Autodesk Fusion 360 part; units mm, degrees
note: some values were not read from the file. Set by a fixed rule: which sketch regions a step uses.
(part 2 of 4)
  line L1067 (-99, -2.5) -> (-101, -2.5)
  line L1068 (-111, -5) -> (-109, -5)
  line L1069 (-109, -5) -> (-109, -2.5)
  line L1070 (-111, -2.5) -> (-111, -5)
  line L1071 (-109, -2.5) -> (-111, -2.5)
  line L1072 (-121, -5) -> (-119, -5)
  line L1073 (-119, -5) -> (-119, -2.5)
  line L1074 (-121, -2.5) -> (-121, -5)
  line L1075 (-119, -2.5) -> (-121, -2.5)
  line L1076 (-131, -5) -> (-129, -5)
  line L1077 (-129, -5) -> (-129, -2.5)
  line L1078 (-131, -2.5) -> (-131, -5)
  line L1079 (-129, -2.5) -> (-131, -2.5)
  line L1080 (-141, -5) -> (-139, -5)
  line L1081 (-139, -5) -> (-139, -2.5)
  line L1082 (-141, -2.5) -> (-141, -5)
  line L1083 (-139, -2.5) -> (-141, -2.5)
  line L1084 (-151, -5) -> (-149, -5)
  line L1085 (-149, -5) -> (-149, -2.5)
  line L1086 (-151, -2.5) -> (-151, -5)
  line L1087 (-149, -2.5) -> (-151, -2.5)
  line L1088 (-11, -15) -> (-9, -15)
  line L1089 (-9, -15) -> (-9, -12.5)
  line L1090 (-11, -12.5) -> (-11, -15)
  line L1091 (-9, -12.5) -> (-11, -12.5)
  line L1092 (-21, -15) -> (-19, -15)
  line L1093 (-19, -15) -> (-19, -12.5)
  line L1094 (-21, -12.5) -> (-21, -15)
  line L1095 (-19, -12.5) -> (-21, -12.5)
  line L1096 (-31, -15) -> (-29, -15)
  line L1097 (-29, -15) -> (-29, -12.5)
  line L1098 (-31, -12.5) -> (-31, -15)
  line L1099 (-29, -12.5) -> (-31, -12.5)
  line L1100 (-41, -15) -> (-39, -15)
  line L1101 (-39, -15) -> (-39, -12.5)
  line L1102 (-41, -12.5) -> (-41, -15)
  line L1103 (-39, -12.5) -> (-41, -12.5)
  line L1104 (-51, -15) -> (-49, -15)
  line L1105 (-49, -15) -> (-49, -12.5)
  line L1106 (-51, -12.5) -> (-51, -15)
  line L1107 (-49, -12.5) -> (-51, -12.5)
  line L1108 (-61, -15) -> (-59, -15)
  line L1109 (-59, -15) -> (-59, -12.5)
  line L1110 (-61, -12.5) -> (-61, -15)
  line L1111 (-59, -12.5) -> (-61, -12.5)
  line L1112 (-71, -15) -> (-69, -15)
  line L1113 (-69, -15) -> (-69, -12.5)
  line L1114 (-71, -12.5) -> (-71, -15)
  line L1115 (-69, -12.5) -> (-71, -12.5)
  line L1116 (-81, -15) -> (-79, -15)
  line L1117 (-79, -15) -> (-79, -12.5)
  line L1118 (-81, -12.5) -> (-81, -15)
  line L1119 (-79, -12.5) -> (-81, -12.5)
  line L1120 (-91, -15) -> (-89, -15)
  line L1121 (-89, -15) -> (-89, -12.5)
  line L1122 (-91, -12.5) -> (-91, -15)
  line L1123 (-89, -12.5) -> (-91, -12.5)
  line L1124 (-101, -15) -> (-99, -15)
  line L1125 (-99, -15) -> (-99, -12.5)
  line L1126 (-101, -12.5) -> (-101, -15)
  line L1127 (-99, -12.5) -> (-101, -12.5)
  line L1128 (-111, -15) -> (-109, -15)
  line L1129 (-109, -15) -> (-109, -12.5)
  line L1130 (-111, -12.5) -> (-111, -15)
  line L1131 (-109, -12.5) -> (-111, -12.5)
  line L1132 (-121, -15) -> (-119, -15)
  line L1133 (-119, -15) -> (-119, -12.5)
  line L1134 (-121, -12.5) -> (-121, -15)
  line L1135 (-119, -12.5) -> (-121, -12.5)
  line L1136 (-131, -15) -> (-129, -15)
  line L1137 (-129, -15) -> (-129, -12.5)
  line L1138 (-131, -12.5) -> (-131, -15)
  line L1139 (-129, -12.5) -> (-131, -12.5)
  line L1140 (-141, -15) -> (-139, -15)
  line L1141 (-139, -15) -> (-139, -12.5)
  line L1142 (-141, -12.5) -> (-141, -15)
  line L1143 (-139, -12.5) -> (-141, -12.5)
  line L1144 (-151, -15) -> (-149, -15)
  line L1145 (-149, -15) -> (-149, -12.5)
  line L1146 (-151, -12.5) -> (-151, -15)
  line L1147 (-149, -12.5) -> (-151, -12.5)
  line L1148 (-11, -25) -> (-9, -25)
  line L1149 (-9, -25) -> (-9, -22.5)
  line L1150 (-11, -22.5) -> (-11, -25)
  line L1151 (-9, -22.5) -> (-11, -22.5)
  line L1152 (-21, -25) -> (-19, -25)
  line L1153 (-19, -25) -> (-19, -22.5)
  line L1154 (-21, -22.5) -> (-21, -25)
  line L1155 (-19, -22.5) -> (-21, -22.5)
  line L1156 (-31, -25) -> (-29, -25)
  line L1157 (-29, -25) -> (-29, -22.5)
  line L1158 (-31, -22.5) -> (-31, -25)
  line L1159 (-29, -22.5) -> (-31, -22.5)
  line L1160 (-41, -25) -> (-39, -25)
  line L1161 (-39, -25) -> (-39, -22.5)
  line L1162 (-41, -22.5) -> (-41, -25)
  line L1163 (-39, -22.5) -> (-41, -22.5)
  line L1164 (-51, -25) -> (-49, -25)
  line L1165 (-49, -25) -> (-49, -22.5)
  line L1166 (-51, -22.5) -> (-51, -25)
  line L1167 (-49, -22.5) -> (-51, -22.5)
  line L1168 (-61, -25) -> (-59, -25)
  line L1169 (-59, -25) -> (-59, -22.5)
  line L1170 (-61, -22.5) -> (-61, -25)
  line L1171 (-59, -22.5) -> (-61, -22.5)
  line L1172 (-71, -25) -> (-69, -25)
  line L1173 (-69, -25) -> (-69, -22.5)
  line L1174 (-71, -22.5) -> (-71, -25)
  line L1175 (-69, -22.5) -> (-71, -22.5)
  line L1176 (-81, -25) -> (-79, -25)
  line L1177 (-79, -25) -> (-79, -22.5)
  line L1178 (-81, -22.5) -> (-81, -25)
  line L1179 (-79, -22.5) -> (-81, -22.5)
  line L1180 (-91, -25) -> (-89, -25)
  line L1181 (-89, -25) -> (-89, -22.5)
  line L1182 (-91, -22.5) -> (-91, -25)
  line L1183 (-89, -22.5) -> (-91, -22.5)
  line L1184 (-101, -25) -> (-99, -25)
  line L1185 (-99, -25) -> (-99, -22.5)
  line L1186 (-101, -22.5) -> (-101, -25)
  line L1187 (-99, -22.5) -> (-101, -22.5)
  line L1188 (-111, -25) -> (-109, -25)
  line L1189 (-109, -25) -> (-109, -22.5)
  line L1190 (-111, -22.5) -> (-111, -25)
  line L1191 (-109, -22.5) -> (-111, -22.5)
  line L1192 (-121, -25) -> (-119, -25)
  line L1193 (-119, -25) -> (-119, -22.5)
  line L1194 (-121, -22.5) -> (-121, -25)
  line L1195 (-119, -22.5) -> (-121, -22.5)
  line L1196 (-131, -25) -> (-129, -25)
  line L1197 (-129, -25) -> (-129, -22.5)
  line L1198 (-131, -22.5) -> (-131, -25)
  line L1199 (-129, -22.5) -> (-131, -22.5)
  line L1200 (-141, -25) -> (-139, -25)
  line L1201 (-139, -25) -> (-139, -22.5)
  line L1202 (-141, -22.5) -> (-141, -25)
  line L1203 (-139, -22.5) -> (-141, -22.5)
  line L1204 (-151, -25) -> (-149, -25)
  line L1205 (-149, -25) -> (-149, -22.5)
  line L1206 (-151, -22.5) -> (-151, -25)
  line L1207 (-149, -22.5) -> (-151, -22.5)
  line L1208 (-11, -35) -> (-9, -35)
  line L1209 (-9, -35) -> (-9, -32.5)
  line L1210 (-11, -32.5) -> (-11, -35)
  line L1211 (-9, -32.5) -> (-11, -32.5)
  line L1212 (-21, -35) -> (-19, -35)
  line L1213 (-19, -35) -> (-19, -32.5)
  line L1214 (-21, -32.5) -> (-21, -35)
  line L1215 (-19, -32.5) -> (-21, -32.5)
  line L1216 (-31, -35) -> (-29, -35)
  line L1217 (-29, -35) -> (-29, -32.5)
  line L1218 (-31, -32.5) -> (-31, -35)
  line L1219 (-29, -32.5) -> (-31, -32.5)
  line L1220 (-41, -35) -> (-39, -35)
  line L1221 (-39, -35) -> (-39, -32.5)
  line L1222 (-41, -32.5) -> (-41, -35)
  line L1223 (-39, -32.5) -> (-41, -32.5)
  line L1224 (-51, -35) -> (-49, -35)
  line L1225 (-49, -35) -> (-49, -32.5)
  line L1226 (-51, -32.5) -> (-51, -35)
  line L1227 (-49, -32.5) -> (-51, -32.5)
  line L1228 (-61, -35) -> (-59, -35)
  line L1229 (-59, -35) -> (-59, -32.5)
  line L1230 (-61, -32.5) -> (-61, -35)
  line L1231 (-59, -32.5) -> (-61, -32.5)
  line L1232 (-71, -35) -> (-69, -35)
  line L1233 (-69, -35) -> (-69, -32.5)
  line L1234 (-71, -32.5) -> (-71, -35)
  line L1235 (-69, -32.5) -> (-71, -32.5)
  line L1236 (-81, -35) -> (-79, -35)
  line L1237 (-79, -35) -> (-79, -32.5)
  line L1238 (-81, -32.5) -> (-81, -35)
  line L1239 (-79, -32.5) -> (-81, -32.5)
  line L1240 (-91, -35) -> (-89, -35)
  line L1241 (-89, -35) -> (-89, -32.5)
  line L1242 (-91, -32.5) -> (-91, -35)
  line L1243 (-89, -32.5) -> (-91, -32.5)
  line L1244 (-101, -35) -> (-99, -35)
  line L1245 (-99, -35) -> (-99, -32.5)
  line L1246 (-101, -32.5) -> (-101, -35)
  line L1247 (-99, -32.5) -> (-101, -32.5)
  line L1248 (-111, -35) -> (-109, -35)
  line L1249 (-109, -35) -> (-109, -32.5)
  line L1250 (-111, -32.5) -> (-111, -35)
  line L1251 (-109, -32.5) -> (-111, -32.5)
  line L1252 (-121, -35) -> (-119, -35)
  line L1253 (-119, -35) -> (-119, -32.5)
  line L1254 (-121, -32.5) -> (-121, -35)
  line L1255 (-119, -32.5) -> (-121, -32.5)
  line L1256 (-131, -35) -> (-129, -35)
  line L1257 (-129, -35) -> (-129, -32.5)
  line L1258 (-131, -32.5) -> (-131, -35)
  line L1259 (-129, -32.5) -> (-131, -32.5)
  line L1260 (-141, -35) -> (-139, -35)
  line L1261 (-139, -35) -> (-139, -32.5)
  line L1262 (-141, -32.5) -> (-141, -35)
  line L1263 (-139, -32.5) -> (-141, -32.5)
  line L1264 (-151, -35) -> (-149, -35)
  line L1265 (-149, -35) -> (-149, -32.5)
  line L1266 (-151, -32.5) -> (-151, -35)
  line L1267 (-149, -32.5) -> (-151, -32.5)
  line L1268 (-11, -45) -> (-9, -45)
  line L1269 (-9, -45) -> (-9, -42.5)
  line L1270 (-11, -42.5) -> (-11, -45)
  line L1271 (-9, -42.5) -> (-11, -42.5)
  line L1272 (-21, -45) -> (-19, -45)
  line L1273 (-19, -45) -> (-19, -42.5)
  line L1274 (-21, -42.5) -> (-21, -45)
  line L1275 (-19, -42.5) -> (-21, -42.5)
  line L1276 (-31, -45) -> (-29, -45)
  line L1277 (-29, -45) -> (-29, -42.5)
  line L1278 (-31, -42.5) -> (-31, -45)
  line L1279 (-29, -42.5) -> (-31, -42.5)
  line L1280 (-41, -45) -> (-39, -45)
  line L1281 (-39, -45) -> (-39, -42.5)
  line L1282 (-41, -42.5) -> (-41, -45)
  line L1283 (-39, -42.5) -> (-41, -42.5)
  line L1284 (-51, -45) -> (-49, -45)
  line L1285 (-49, -45) -> (-49, -42.5)
  line L1286 (-51, -42.5) -> (-51, -45)
  line L1287 (-49, -42.5) -> (-51, -42.5)
  line L1288 (-61, -45) -> (-59, -45)
  line L1289 (-59, -45) -> (-59, -42.5)
  line L1290 (-61, -42.5) -> (-61, -45)
  line L1291 (-59, -42.5) -> (-61, -42.5)
  line L1292 (-71, -45) -> (-69, -45)
  line L1293 (-69, -45) -> (-69, -42.5)
  line L1294 (-71, -42.5) -> (-71, -45)
  line L1295 (-69, -42.5) -> (-71, -42.5)
  line L1296 (-81, -45) -> (-79, -45)
  line L1297 (-79, -45) -> (-79, -42.5)
  line L1298 (-81, -42.5) -> (-81, -45)
  line L1299 (-79, -42.5) -> (-81, -42.5)
  line L1300 (-91, -45) -> (-89, -45)
  line L1301 (-89, -45) -> (-89, -42.5)
  line L1302 (-91, -42.5) -> (-91, -45)
  line L1303 (-89, -42.5) -> (-91, -42.5)
  line L1304 (-101, -45) -> (-99, -45)
  line L1305 (-99, -45) -> (-99, -42.5)
  line L1306 (-101, -42.5) -> (-101, -45)
  line L1307 (-99, -42.5) -> (-101, -42.5)
  line L1308 (-111, -45) -> (-109, -45)
  line L1309 (-109, -45) -> (-109, -42.5)
  line L1310 (-111, -42.5) -> (-111, -45)
  line L1311 (-109, -42.5) -> (-111, -42.5)
  line L1312 (-121, -45) -> (-119, -45)
  line L1313 (-119, -45) -> (-119, -42.5)
  line L1314 (-121, -42.5) -> (-121, -45)
  line L1315 (-119, -42.5) -> (-121, -42.5)
  line L1316 (-131, -45) -> (-129, -45)
  line L1317 (-129, -45) -> (-129, -42.5)
  line L1318 (-131, -42.5) -> (-131, -45)
  line L1319 (-129, -42.5) -> (-131, -42.5)
  line L1320 (-141, -45) -> (-139, -45)
  line L1321 (-139, -45) -> (-139, -42.5)
  line L1322 (-141, -42.5) -> (-141, -45)
  line L1323 (-139, -42.5) -> (-141, -42.5)
  line L1324 (-151, -45) -> (-149, -45)
  line L1325 (-149, -45) -> (-149, -42.5)
  line L1326 (-151, -42.5) -> (-151, -45)
  line L1327 (-149, -42.5) -> (-151, -42.5)
  line L1328 (-11, -55) -> (-9, -55)
  line L1329 (-9, -55) -> (-9, -52.5)
  line L1330 (-11, -52.5) -> (-11, -55)
  line L1331 (-9, -52.5) -> (-11, -52.5)
  line L1332 (-21, -55) -> (-19, -55)
  line L1333 (-19, -55) -> (-19, -52.5)
  line L1334 (-21, -52.5) -> (-21, -55)
  line L1335 (-19, -52.5) -> (-21, -52.5)
  line L1336 (-31, -55) -> (-29, -55)
  line L1337 (-29, -55) -> (-29, -52.5)
  line L1338 (-31, -52.5) -> (-31, -55)
  line L1339 (-29, -52.5) -> (-31, -52.5)
  line L1340 (-41, -55) -> (-39, -55)
  line L1341 (-39, -55) -> (-39, -52.5)
  line L1342 (-41, -52.5) -> (-41, -55)
  line L1343 (-39, -52.5) -> (-41, -52.5)
  line L1344 (-51, -55) -> (-49, -55)
  line L1345 (-49, -55) -> (-49, -52.5)
  line L1346 (-51, -52.5) -> (-51, -55)
  line L1347 (-49, -52.5) -> (-51, -52.5)
  line L1348 (-61, -55) -> (-59, -55)
  line L1349 (-59, -55) -> (-59, -52.5)
  line L1350 (-61, -52.5) -> (-61, -55)
  line L1351 (-59, -52.5) -> (-61, -52.5)
  line L1352 (-71, -55) -> (-69, -55)
  line L1353 (-69, -55) -> (-69, -52.5)
  line L1354 (-71, -52.5) -> (-71, -55)
  line L1355 (-69, -52.5) -> (-71, -52.5)
  line L1356 (-81, -55) -> (-79, -55)
  line L1357 (-79, -55) -> (-79, -52.5)
  line L1358 (-81, -52.5) -> (-81, -55)
  line L1359 (-79, -52.5) -> (-81, -52.5)
  line L1360 (-91, -55) -> (-89, -55)
  line L1361 (-89, -55) -> (-89, -52.5)
  line L1362 (-91, -52.5) -> (-91, -55)
  line L1363 (-89, -52.5) -> (-91, -52.5)
  line L1364 (-101, -55) -> (-99, -55)
  line L1365 (-99, -55) -> (-99, -52.5)
  line L1366 (-101, -52.5) -> (-101, -55)
  line L1367 (-99, -52.5) -> (-101, -52.5)
  line L1368 (-111, -55) -> (-109, -55)
  line L1369 (-109, -55) -> (-109, -52.5)
  line L1370 (-111, -52.5) -> (-111, -55)
  line L1371 (-109, -52.5) -> (-111, -52.5)
  line L1372 (-121, -55) -> (-119, -55)
  line L1373 (-119, -55) -> (-119, -52.5)
  line L1374 (-121, -52.5) -> (-121, -55)
  line L1375 (-119, -52.5) -> (-121, -52.5)
  line L1376 (-131, -55) -> (-129, -55)
  line L1377 (-129, -55) -> (-129, -52.5)
  line L1378 (-131, -52.5) -> (-131, -55)
  line L1379 (-129, -52.5) -> (-131, -52.5)
  line L1380 (-141, -55) -> (-139, -55)
  line L1381 (-139, -55) -> (-139, -52.5)
  line L1382 (-141, -52.5) -> (-141, -55)
  line L1383 (-139, -52.5) -> (-141, -52.5)
  line L1384 (-151, -55) -> (-149, -55)
  line L1385 (-149, -55) -> (-149, -52.5)
  line L1386 (-151, -52.5) -> (-151, -55)
  line L1387 (-149, -52.5) -> (-151, -52.5)
  line L1388 (-11, -65) -> (-9, -65)
  line L1389 (-9, -65) -> (-9, -62.5)
  line L1390 (-11, -62.5) -> (-11, -65)
  line L1391 (-9, -62.5) -> (-11, -62.5)
  line L1392 (-21, -65) -> (-19, -65)
  line L1393 (-19, -65) -> (-19, -62.5)
  line L1394 (-21, -62.5) -> (-21, -65)
  line L1395 (-19, -62.5) -> (-21, -62.5)
  line L1396 (-31, -65) -> (-29, -65)
  line L1397 (-29, -65) -> (-29, -62.5)
  line L1398 (-31, -62.5) -> (-31, -65)
  line L1399 (-29, -62.5) -> (-31, -62.5)
  line L1400 (-41, -65) -> (-39, -65)
  line L1401 (-39, -65) -> (-39, -62.5)
  line L1402 (-41, -62.5) -> (-41, -65)
  line L1403 (-39, -62.5) -> (-41, -62.5)
  line L1404 (-51, -65) -> (-49, -65)
  line L1405 (-49, -65) -> (-49, -62.5)
  line L1406 (-51, -62.5) -> (-51, -65)
  line L1407 (-49, -62.5) -> (-51, -62.5)
  line L1408 (-61, -65) -> (-59, -65)
  line L1409 (-59, -65) -> (-59, -62.5)
  line L1410 (-61, -62.5) -> (-61, -65)
  line L1411 (-59, -62.5) -> (-61, -62.5)
  line L1412 (-71, -65) -> (-69, -65)
  line L1413 (-69, -65) -> (-69, -62.5)
  line L1414 (-71, -62.5) -> (-71, -65)
  line L1415 (-69, -62.5) -> (-71, -62.5)
  line L1416 (-81, -65) -> (-79, -65)
  line L1417 (-79, -65) -> (-79, -62.5)
  line L1418 (-81, -62.5) -> (-81, -65)
  line L1419 (-79, -62.5) -> (-81, -62.5)
  line L1420 (-91, -65) -> (-89, -65)
  line L1421 (-89, -65) -> (-89, -62.5)
  line L1422 (-91, -62.5) -> (-91, -65)
  line L1423 (-89, -62.5) -> (-91, -62.5)
  line L1424 (-101, -65) -> (-99, -65)
  line L1425 (-99, -65) -> (-99, -62.5)
  line L1426 (-101, -62.5) -> (-101, -65)
  line L1427 (-99, -62.5) -> (-101, -62.5)
  line L1428 (-111, -65) -> (-109, -65)
  line L1429 (-109, -65) -> (-109, -62.5)
  line L1430 (-111, -62.5) -> (-111, -65)
  line L1431 (-109, -62.5) -> (-111, -62.5)
  line L1432 (-121, -65) -> (-119, -65)
  line L1433 (-119, -65) -> (-119, -62.5)
  line L1434 (-121, -62.5) -> (-121, -65)
  line L1435 (-119, -62.5) -> (-121, -62.5)
  line L1436 (-131, -65) -> (-129, -65)
  line L1437 (-129, -65) -> (-129, -62.5)
  line L1438 (-131, -62.5) -> (-131, -65)
  line L1439 (-129, -62.5) -> (-131, -62.5)
  line L1440 (-141, -65) -> (-139, -65)
  line L1441 (-139, -65) -> (-139, -62.5)
  line L1442 (-141, -62.5) -> (-141, -65)
  line L1443 (-139, -62.5) -> (-141, -62.5)
  line L1444 (-151, -65) -> (-149, -65)
  line L1445 (-149, -65) -> (-149, -62.5)
  line L1446 (-151, -62.5) -> (-151, -65)
  line L1447 (-149, -62.5) -> (-151, -62.5)
  line L1448 (-11, -75) -> (-9, -75)
  line L1449 (-9, -75) -> (-9, -72.5)
  line L1450 (-11, -72.5) -> (-11, -75)
  line L1451 (-9, -72.5) -> (-11, -72.5)
  line L1452 (-21, -75) -> (-19, -75)
  line L1453 (-19, -75) -> (-19, -72.5)
  line L1454 (-21, -72.5) -> (-21, -75)
  line L1455 (-19, -72.5) -> (-21, -72.5)
  line L1456 (-31, -75) -> (-29, -75)
  line L1457 (-29, -75) -> (-29, -72.5)
  line L1458 (-31, -72.5) -> (-31, -75)
  line L1459 (-29, -72.5) -> (-31, -72.5)
  line L1460 (-41, -75) -> (-39, -75)
  line L1461 (-39, -75) -> (-39, -72.5)
  line L1462 (-41, -72.5) -> (-41, -75)
  line L1463 (-39, -72.5) -> (-41, -72.5)
  line L1464 (-51, -75) -> (-49, -75)
  line L1465 (-49, -75) -> (-49, -72.5)
  line L1466 (-51, -72.5) -> (-51, -75)
  line L1467 (-49, -72.5) -> (-51, -72.5)
  line L1468 (-61, -75) -> (-59, -75)
  line L1469 (-59, -75) -> (-59, -72.5)
  line L1470 (-61, -72.5) -> (-61, -75)
  line L1471 (-59, -72.5) -> (-61, -72.5)
  line L1472 (-71, -75) -> (-69, -75)
  line L1473 (-69, -75) -> (-69, -72.5)
  line L1474 (-71, -72.5) -> (-71, -75)
  line L1475 (-69, -72.5) -> (-71, -72.5)
  line L1476 (-81, -75) -> (-79, -75)
  line L1477 (-79, -75) -> (-79, -72.5)
  line L1478 (-81, -72.5) -> (-81, -75)
  line L1479 (-79, -72.5) -> (-81, -72.5)
  line L1480 (-91, -75) -> (-89, -75)
  line L1481 (-89, -75) -> (-89, -72.5)
  line L1482 (-91, -72.5) -> (-91, -75)
  line L1483 (-89, -72.5) -> (-91, -72.5)
  line L1484 (-101, -75) -> (-99, -75)
  line L1485 (-99, -75) -> (-99, -72.5)
  line L1486 (-101, -72.5) -> (-101, -75)
  line L1487 (-99, -72.5) -> (-101, -72.5)
  line L1488 (-111, -75) -> (-109, -75)
  line L1489 (-109, -75) -> (-109, -72.5)
  line L1490 (-111, -72.5) -> (-111, -75)
  line L1491 (-109, -72.5) -> (-111, -72.5)
  line L1492 (-121, -75) -> (-119, -75)
  line L1493 (-119, -75) -> (-119, -72.5)
  line L1494 (-121, -72.5) -> (-121, -75)
  line L1495 (-119, -72.5) -> (-121, -72.5)
  line L1496 (-131, -75) -> (-129, -75)
  line L1497 (-129, -75) -> (-129, -72.5)
  line L1498 (-131, -72.5) -> (-131, -75)
  line L1499 (-129, -72.5) -> (-131, -72.5)
  line L1500 (-141, -75) -> (-139, -75)
  line L1501 (-139, -75) -> (-139, -72.5)
  line L1502 (-141, -72.5) -> (-141, -75)
  line L1503 (-139, -72.5) -> (-141, -72.5)
  line L1504 (-151, -75) -> (-149, -75)
  line L1505 (-149, -75) -> (-149, -72.5)
  line L1506 (-151, -72.5) -> (-151, -75)
  line L1507 (-149, -72.5) -> (-151, -72.5)
  line L1508 (-11, -85) -> (-9, -85)
  line L1509 (-9, -85) -> (-9, -82.5)
  line L1510 (-11, -82.5) -> (-11, -85)
  line L1511 (-9, -82.5) -> (-11, -82.5)
  line L1512 (-21, -85) -> (-19, -85)
  line L1513 (-19, -85) -> (-19, -82.5)
  line L1514 (-21, -82.5) -> (-21, -85)
  line L1515 (-19, -82.5) -> (-21, -82.5)
  line L1516 (-31, -85) -> (-29, -85)
  line L1517 (-29, -85) -> (-29, -82.5)
  line L1518 (-31, -82.5) -> (-31, -85)
  line L1519 (-29, -82.5) -> (-31, -82.5)
  line L1520 (-41, -85) -> (-39, -85)
  line L1521 (-39, -85) -> (-39, -82.5)
  line L1522 (-41, -82.5) -> (-41, -85)
  line L1523 (-39, -82.5) -> (-41, -82.5)
  line L1524 (-51, -85) -> (-49, -85)
  line L1525 (-49, -85) -> (-49, -82.5)
  line L1526 (-51, -82.5) -> (-51, -85)
  line L1527 (-49, -82.5) -> (-51, -82.5)
  line L1528 (-61, -85) -> (-59, -85)
  line L1529 (-59, -85) -> (-59, -82.5)
  line L1530 (-61, -82.5) -> (-61, -85)
  line L1531 (-59, -82.5) -> (-61, -82.5)
  line L1532 (-71, -85) -> (-69, -85)
  line L1533 (-69, -85) -> (-69, -82.5)
  line L1534 (-71, -82.5) -> (-71, -85)
  line L1535 (-69, -82.5) -> (-71, -82.5)
  line L1536 (-81, -85) -> (-79, -85)
  line L1537 (-79, -85) -> (-79, -82.5)
  line L1538 (-81, -82.5) -> (-81, -85)
  line L1539 (-79, -82.5) -> (-81, -82.5)
  line L1540 (-91, -85) -> (-89, -85)
  line L1541 (-89, -85) -> (-89, -82.5)
  line L1542 (-91, -82.5) -> (-91, -85)
  line L1543 (-89, -82.5) -> (-91, -82.5)
  line L1544 (-101, -85) -> (-99, -85)
  line L1545 (-99, -85) -> (-99, -82.5)
  line L1546 (-101, -82.5) -> (-101, -85)
  line L1547 (-99, -82.5) -> (-101, -82.5)
  line L1548 (-111, -85) -> (-109, -85)
  line L1549 (-109, -85) -> (-109, -82.5)
  line L1550 (-111, -82.5) -> (-111, -85)
  line L1551 (-109, -82.5) -> (-111, -82.5)
  line L1552 (-121, -85) -> (-119, -85)
  line L1553 (-119, -85) -> (-119, -82.5)
  line L1554 (-121, -82.5) -> (-121, -85)
  line L1555 (-119, -82.5) -> (-121, -82.5)
  line L1556 (-131, -85) -> (-129, -85)
  line L1557 (-129, -85) -> (-129, -82.5)
  line L1558 (-131, -82.5) -> (-131, -85)
  line L1559 (-129, -82.5) -> (-131, -82.5)
  line L1560 (-141, -85) -> (-139, -85)
  line L1561 (-139, -85) -> (-139, -82.5)
  line L1562 (-141, -82.5) -> (-141, -85)
  line L1563 (-139, -82.5) -> (-141, -82.5)
  line L1564 (-151, -85) -> (-149, -85)
  line L1565 (-149, -85) -> (-149, -82.5)
  line L1566 (-151, -82.5) -> (-151, -85)
  line L1567 (-149, -82.5) -> (-151, -82.5)
  line L1568 (-11, -95) -> (-9, -95)
  line L1569 (-9, -95) -> (-9, -92.5)
  line L1570 (-11, -92.5) -> (-11, -95)
  line L1571 (-9, -92.5) -> (-11, -92.5)
  line L1572 (-21, -95) -> (-19, -95)
  line L1573 (-19, -95) -> (-19, -92.5)
  line L1574 (-21, -92.5) -> (-21, -95)
  line L1575 (-19, -92.5) -> (-21, -92.5)
  line L1576 (-31, -95) -> (-29, -95)
  line L1577 (-29, -95) -> (-29, -92.5)
  line L1578 (-31, -92.5) -> (-31, -95)
  line L1579 (-29, -92.5) -> (-31, -92.5)
  line L1580 (-41, -95) -> (-39, -95)
  line L1581 (-39, -95) -> (-39, -92.5)
  line L1582 (-41, -92.5) -> (-41, -95)
  line L1583 (-39, -92.5) -> (-41, -92.5)
  line L1584 (-51, -95) -> (-49, -95)
  line L1585 (-49, -95) -> (-49, -92.5)
  line L1586 (-51, -92.5) -> (-51, -95)
  line L1587 (-49, -92.5) -> (-51, -92.5)
  line L1588 (-61, -95) -> (-59, -95)
  line L1589 (-59, -95) -> (-59, -92.5)
  line L1590 (-61, -92.5) -> (-61, -95)
  line L1591 (-59, -92.5) -> (-61, -92.5)
  line L1592 (-71, -95) -> (-69, -95)
  line L1593 (-69, -95) -> (-69, -92.5)
  line L1594 (-71, -92.5) -> (-71, -95)
  line L1595 (-69, -92.5) -> (-71, -92.5)
  line L1596 (-81, -95) -> (-79, -95)
  line L1597 (-79, -95) -> (-79, -92.5)
  line L1598 (-81, -92.5) -> (-81, -95)
  line L1599 (-79, -92.5) -> (-81, -92.5)
  line L1600 (-91, -95) -> (-89, -95)
  line L1601 (-89, -95) -> (-89, -92.5)
  line L1602 (-91, -92.5) -> (-91, -95)
  line L1603 (-89, -92.5) -> (-91, -92.5)
  line L1604 (-101, -95) -> (-99, -95)
  line L1605 (-99, -95) -> (-99, -92.5)
  line L1606 (-101, -92.5) -> (-101, -95)
  line L1607 (-99, -92.5) -> (-101, -92.5)
  line L1608 (-111, -95) -> (-109, -95)
  line L1609 (-109, -95) -> (-109, -92.5)
  line L1610 (-111, -92.5) -> (-111, -95)
  line L1611 (-109, -92.5) -> (-111, -92.5)
  line L1612 (-121, -95) -> (-119, -95)
  line L1613 (-119, -95) -> (-119, -92.5)
  line L1614 (-121, -92.5) -> (-121, -95)
  line L1615 (-119, -92.5) -> (-121, -92.5)
  line L1616 (-131, -95) -> (-129, -95)
  line L1617 (-129, -95) -> (-129, -92.5)
  line L1618 (-131, -92.5) -> (-131, -95)
  line L1619 (-129, -92.5) -> (-131, -92.5)
  line L1620 (-141, -95) -> (-139, -95)
  line L1621 (-139, -95) -> (-139, -92.5)
  line L1622 (-141, -92.5) -> (-141, -95)
  line L1623 (-139, -92.5) -> (-141, -92.5)
  line L1624 (-151, -95) -> (-149, -95)
  line L1625 (-149, -95) -> (-149, -92.5)
  line L1626 (-151, -92.5) -> (-151, -95)
  line L1627 (-149, -92.5) -> (-151, -92.5)
  line L1628 (-11, -105) -> (-9, -105)
  line L1629 (-9, -105) -> (-9, -102.5)
  line L1630 (-11, -102.5) -> (-11, -105)
  line L1631 (-9, -102.5) -> (-11, -102.5)
  line L1632 (-21, -105) -> (-19, -105)
  line L1633 (-19, -105) -> (-19, -102.5)
  line L1634 (-21, -102.5) -> (-21, -105)
  line L1635 (-19, -102.5) -> (-21, -102.5)
  line L1636 (-31, -105) -> (-29, -105)
  line L1637 (-29, -105) -> (-29, -102.5)
  line L1638 (-31, -102.5) -> (-31, -105)
  line L1639 (-29, -102.5) -> (-31, -102.5)
  line L1640 (-41, -105) -> (-39, -105)
  line L1641 (-39, -105) -> (-39, -102.5)
  line L1642 (-41, -102.5) -> (-41, -105)
  line L1643 (-39, -102.5) -> (-41, -102.5)
  line L1644 (-51, -105) -> (-49, -105)
  line L1645 (-49, -105) -> (-49, -102.5)
  line L1646 (-51, -102.5) -> (-51, -105)
  line L1647 (-49, -102.5) -> (-51, -102.5)
  line L1648 (-61, -105) -> (-59, -105)
  line L1649 (-59, -105) -> (-59, -102.5)
  line L1650 (-61, -102.5) -> (-61, -105)
  line L1651 (-59, -102.5) -> (-61, -102.5)
  line L1652 (-71, -105) -> (-69, -105)
  line L1653 (-69, -105) -> (-69, -102.5)
  line L1654 (-71, -102.5) -> (-71, -105)
  line L1655 (-69, -102.5) -> (-71, -102.5)
  line L1656 (-81, -105) -> (-79, -105)
  line L1657 (-79, -105) -> (-79, -102.5)
  line L1658 (-81, -102.5) -> (-81, -105)
  line L1659 (-79, -102.5) -> (-81, -102.5)
  line L1660 (-91, -105) -> (-89, -105)
  line L1661 (-89, -105) -> (-89, -102.5)
  line L1662 (-91, -102.5) -> (-91, -105)
  line L1663 (-89, -102.5) -> (-91, -102.5)
  line L1664 (-101, -105) -> (-99, -105)
  line L1665 (-99, -105) -> (-99, -102.5)
  line L1666 (-101, -102.5) -> (-101, -105)
  line L1667 (-99, -102.5) -> (-101, -102.5)
  line L1668 (-111, -105) -> (-109, -105)
  line L1669 (-109, -105) -> (-109, -102.5)
  line L1670 (-111, -102.5) -> (-111, -105)
  line L1671 (-109, -102.5) -> (-111, -102.5)
  line L1672 (-121, -105) -> (-119, -105)
  line L1673 (-119, -105) -> (-119, -102.5)
  line L1674 (-121, -102.5) -> (-121, -105)
  line L1675 (-119, -102.5) -> (-121, -102.5)
  line L1676 (-131, -105) -> (-129, -105)
  line L1677 (-129, -105) -> (-129, -102.5)
  line L1678 (-131, -102.5) -> (-131, -105)
  line L1679 (-129, -102.5) -> (-131, -102.5)
  line L1680 (-141, -105) -> (-139, -105)
  line L1681 (-139, -105) -> (-139, -102.5)
  line L1682 (-141, -102.5) -> (-141, -105)
  line L1683 (-139, -102.5) -> (-141, -102.5)
  line L1684 (-151, -105) -> (-149, -105)
  line L1685 (-149, -105) -> (-149, -102.5)
  line L1686 (-151, -102.5) -> (-151, -105)
  line L1687 (-149, -102.5) -> (-151, -102.5)
  line L1688 (-11, -115) -> (-9, -115)
  line L1689 (-9, -115) -> (-9, -112.5)
  line L1690 (-11, -112.5) -> (-11, -115)
  line L1691 (-9, -112.5) -> (-11, -112.5)
  line L1692 (-21, -115) -> (-19, -115)
  line L1693 (-19, -115) -> (-19, -112.5)
  line L1694 (-21, -112.5) -> (-21, -115)
  line L1695 (-19, -112.5) -> (-21, -112.5)
  line L1696 (-31, -115) -> (-29, -115)
  line L1697 (-29, -115) -> (-29, -112.5)
  line L1698 (-31, -112.5) -> (-31, -115)
  line L1699 (-29, -112.5) -> (-31, -112.5)
  line L1700 (-41, -115) -> (-39, -115)
  line L1701 (-39, -115) -> (-39, -112.5)
  line L1702 (-41, -112.5) -> (-41, -115)
  line L1703 (-39, -112.5) -> (-41, -112.5)
  line L1704 (-51, -115) -> (-49, -115)
  line L1705 (-49, -115) -> (-49, -112.5)
  line L1706 (-51, -112.5) -> (-51, -115)
  line L1707 (-49, -112.5) -> (-51, -112.5)
  line L1708 (-61, -115) -> (-59, -115)
  line L1709 (-59, -115) -> (-59, -112.5)
  line L1710 (-61, -112.5) -> (-61, -115)
  line L1711 (-59, -112.5) -> (-61, -112.5)
  line L1712 (-71, -115) -> (-69, -115)
  line L1713 (-69, -115) -> (-69, -112.5)
  line L1714 (-71, -112.5) -> (-71, -115)
  line L1715 (-69, -112.5) -> (-71, -112.5)
  line L1716 (-81, -115) -> (-79, -115)
  line L1717 (-79, -115) -> (-79, -112.5)
  line L1718 (-81, -112.5) -> (-81, -115)
  line L1719 (-79, -112.5) -> (-81, -112.5)
  line L1720 (-91, -115) -> (-89, -115)
  line L1721 (-89, -115) -> (-89, -112.5)
  line L1722 (-91, -112.5) -> (-91, -115)
  line L1723 (-89, -112.5) -> (-91, -112.5)
  line L1724 (-101, -115) -> (-99, -115)
  line L1725 (-99, -115) -> (-99, -112.5)
  line L1726 (-101, -112.5) -> (-101, -115)
  line L1727 (-99, -112.5) -> (-101, -112.5)
  line L1728 (-111, -115) -> (-109, -115)
  line L1729 (-109, -115) -> (-109, -112.5)
  line L1730 (-111, -112.5) -> (-111, -115)
  line L1731 (-109, -112.5) -> (-111, -112.5)
  line L1732 (-121, -115) -> (-119, -115)
  line L1733 (-119, -115) -> (-119, -112.5)
  line L1734 (-121, -112.5) -> (-121, -115)
  line L1735 (-119, -112.5) -> (-121, -112.5)
  line L1736 (-131, -115) -> (-129, -115)
  line L1737 (-129, -115) -> (-129, -112.5)
  line L1738 (-131, -112.5) -> (-131, -115)
  line L1739 (-129, -112.5) -> (-131, -112.5)
  line L1740 (-141, -115) -> (-139, -115)
  line L1741 (-139, -115) -> (-139, -112.5)
  line L1742 (-141, -112.5) -> (-141, -115)
  line L1743 (-139, -112.5) -> (-141, -112.5)
  line L1744 (-151, -115) -> (-149, -115)
  line L1745 (-149, -115) -> (-149, -112.5)
  line L1746 (-151, -112.5) -> (-151, -115)
  line L1747 (-149, -112.5) -> (-151, -112.5)
  line L1748 (-11, -125) -> (-9, -125)
  line L1749 (-9, -125) -> (-9, -122.5)
  line L1750 (-11, -122.5) -> (-11, -125)
  line L1751 (-9, -122.5) -> (-11, -122.5)
  line L1752 (-21, -125) -> (-19, -125)
  line L1753 (-19, -125) -> (-19, -122.5)
  line L1754 (-21, -122.5) -> (-21, -125)
  line L1755 (-19, -122.5) -> (-21, -122.5)
  line L1756 (-31, -125) -> (-29, -125)
  line L1757 (-29, -125) -> (-29, -122.5)
  line L1758 (-31, -122.5) -> (-31, -125)
  line L1759 (-29, -122.5) -> (-31, -122.5)
  line L1760 (-41, -125) -> (-39, -125)
  line L1761 (-39, -125) -> (-39, -122.5)
  line L1762 (-41, -122.5) -> (-41, -125)
  line L1763 (-39, -122.5) -> (-41, -122.5)
  line L1764 (-51, -125) -> (-49, -125)
  line L1765 (-49, -125) -> (-49, -122.5)
  line L1766 (-51, -122.5) -> (-51, -125)
  line L1767 (-49, -122.5) -> (-51, -122.5)
  line L1768 (-61, -125) -> (-59, -125)
  line L1769 (-59, -125) -> (-59, -122.5)
  line L1770 (-61, -122.5) -> (-61, -125)
  line L1771 (-59, -122.5) -> (-61, -122.5)
  line L1772 (-71, -125) -> (-69, -125)
  line L1773 (-69, -125) -> (-69, -122.5)
  line L1774 (-71, -122.5) -> (-71, -125)
  line L1775 (-69, -122.5) -> (-71, -122.5)
  line L1776 (-81, -125) -> (-79, -125)
  line L1777 (-79, -125) -> (-79, -122.5)
  line L1778 (-81, -122.5) -> (-81, -125)
  line L1779 (-79, -122.5) -> (-81, -122.5)
  line L1780 (-91, -125) -> (-89, -125)
  line L1781 (-89, -125) -> (-89, -122.5)
  line L1782 (-91, -122.5) -> (-91, -125)
  line L1783 (-89, -122.5) -> (-91, -122.5)
  line L1784 (-101, -125) -> (-99, -125)
  line L1785 (-99, -125) -> (-99, -122.5)
  line L1786 (-101, -122.5) -> (-101, -125)
  line L1787 (-99, -122.5) -> (-101, -122.5)
  line L1788 (-111, -125) -> (-109, -125)
  line L1789 (-109, -125) -> (-109, -122.5)
  line L1790 (-111, -122.5) -> (-111, -125)
  line L1791 (-109, -122.5) -> (-111, -122.5)
  line L1792 (-121, -125) -> (-119, -125)
  line L1793 (-119, -125) -> (-119, -122.5)
  line L1794 (-121, -122.5) -> (-121, -125)
  line L1795 (-119, -122.5) -> (-121, -122.5)
  line L1796 (-131, -125) -> (-129, -125)
  line L1797 (-129, -125) -> (-129, -122.5)
  line L1798 (-131, -122.5) -> (-131, -125)
  line L1799 (-129, -122.5) -> (-131, -122.5)
  line L1800 (-141, -125) -> (-139, -125)
  line L1801 (-139, -125) -> (-139, -122.5)
  line L1802 (-141, -122.5) -> (-141, -125)
  line L1803 (-139, -122.5) -> (-141, -122.5)
  line L1804 (-151, -125) -> (-149, -125)
  line L1805 (-149, -125) -> (-149, -122.5)
  line L1806 (-151, -122.5) -> (-151, -125)
  line L1807 (-149, -122.5) -> (-151, -122.5)
  line L1808 (-11, -135) -> (-9, -135)
  line L1809 (-9, -135) -> (-9, -132.5)
  line L1810 (-11, -132.5) -> (-11, -135)
  line L1811 (-9, -132.5) -> (-11, -132.5)
  line L1812 (-21, -135) -> (-19, -135)
  line L1813 (-19, -135) -> (-19, -132.5)
  line L1814 (-21, -132.5) -> (-21, -135)
  line L1815 (-19, -132.5) -> (-21, -132.5)
  line L1816 (-31, -135) -> (-29, -135)
  line L1817 (-29, -135) -> (-29, -132.5)
  line L1818 (-31, -132.5) -> (-31, -135)
  line L1819 (-29, -132.5) -> (-31, -132.5)
  line L1820 (-41, -135) -> (-39, -135)
  line L1821 (-39, -135) -> (-39, -132.5)
  line L1822 (-41, -132.5) -> (-41, -135)
  line L1823 (-39, -132.5) -> (-41, -132.5)
  line L1824 (-51, -135) -> (-49, -135)
  line L1825 (-49, -135) -> (-49, -132.5)
  line L1826 (-51, -132.5) -> (-51, -135)
  line L1827 (-49, -132.5) -> (-51, -132.5)
  line L1828 (-61, -135) -> (-59, -135)
  line L1829 (-59, -135) -> (-59, -132.5)
  line L1830 (-61, -132.5) -> (-61, -135)
  line L1831 (-59, -132.5) -> (-61, -132.5)
  line L1832 (-71, -135) -> (-69, -135)
  line L1833 (-69, -135) -> (-69, -132.5)
  line L1834 (-71, -132.5) -> (-71, -135)
  line L1835 (-69, -132.5) -> (-71, -132.5)
  line L1836 (-81, -135) -> (-79, -135)
  line L1837 (-79, -135) -> (-79, -132.5)
  line L1838 (-81, -132.5) -> (-81, -135)
  line L1839 (-79, -132.5) -> (-81, -132.5)
  line L1840 (-91, -135) -> (-89, -135)
  line L1841 (-89, -135) -> (-89, -132.5)
  line L1842 (-91, -132.5) -> (-91, -135)
  line L1843 (-89, -132.5) -> (-91, -132.5)
  line L1844 (-101, -135) -> (-99, -135)
  line L1845 (-99, -135) -> (-99, -132.5)
  line L1846 (-101, -132.5) -> (-101, -135)
  line L1847 (-99, -132.5) -> (-101, -132.5)
  line L1848 (-111, -135) -> (-109, -135)
  line L1849 (-109, -135) -> (-109, -132.5)
  line L1850 (-111, -132.5) -> (-111, -135)
  line L1851 (-109, -132.5) -> (-111, -132.5)
  line L1852 (-121, -135) -> (-119, -135)
  line L1853 (-119, -135) -> (-119, -132.5)
  line L1854 (-121, -132.5) -> (-121, -135)
  line L1855 (-119, -132.5) -> (-121, -132.5)
  line L1856 (-131, -135) -> (-129, -135)
  line L1857 (-129, -135) -> (-129, -132.5)
  line L1858 (-131, -132.5) -> (-131, -135)
  line L1859 (-129, -132.5) -> (-131, -132.5)
  line L1860 (-141, -135) -> (-139, -135)
  line L1861 (-139, -135) -> (-139, -132.5)
  line L1862 (-141, -132.5) -> (-141, -135)
  line L1863 (-139, -132.5) -> (-141, -132.5)
  line L1864 (-151, -135) -> (-149, -135)
  line L1865 (-149, -135) -> (-149, -132.5)
  line L1866 (-151, -132.5) -> (-151, -135)
  line L1867 (-149, -132.5) -> (-151, -132.5)
  line L1868 (-11, -145) -> (-9, -145)
  line L1869 (-9, -145) -> (-9, -142.5)
  line L1870 (-11, -142.5) -> (-11, -145)
  line L1871 (-9, -142.5) -> (-11, -142.5)
  line L1872 (-21, -145) -> (-19, -145)
  line L1873 (-19, -145) -> (-19, -142.5)
  line L1874 (-21, -142.5) -> (-21, -145)
  line L1875 (-19, -142.5) -> (-21, -142.5)
  line L1876 (-31, -145) -> (-29, -145)
  line L1877 (-29, -145) -> (-29, -142.5)
  line L1878 (-31, -142.5) -> (-31, -145)
  line L1879 (-29, -142.5) -> (-31, -142.5)
  line L1880 (-41, -145) -> (-39, -145)
  line L1881 (-39, -145) -> (-39, -142.5)
  line L1882 (-41, -142.5) -> (-41, -145)
  line L1883 (-39, -142.5) -> (-41, -142.5)
  line L1884 (-51, -145) -> (-49, -145)
  line L1885 (-49, -145) -> (-49, -142.5)
  line L1886 (-51, -142.5) -> (-51, -145)
  line L1887 (-49, -142.5) -> (-51, -142.5)
  line L1888 (-61, -145) -> (-59, -145)
  line L1889 (-59, -145) -> (-59, -142.5)
  line L1890 (-61, -142.5) -> (-61, -145)
  line L1891 (-59, -142.5) -> (-61, -142.5)
  line L1892 (-71, -145) -> (-69, -145)
  line L1893 (-69, -145) -> (-69, -142.5)
  line L1894 (-71, -142.5) -> (-71, -145)
  line L1895 (-69, -142.5) -> (-71, -142.5)
  line L1896 (-81, -145) -> (-79, -145)
  line L1897 (-79, -145) -> (-79, -142.5)
  line L1898 (-81, -142.5) -> (-81, -145)
  line L1899 (-79, -142.5) -> (-81, -142.5)
  line L1900 (-91, -145) -> (-89, -145)
  line L1901 (-89, -145) -> (-89, -142.5)
  line L1902 (-91, -142.5) -> (-91, -145)
  line L1903 (-89, -142.5) -> (-91, -142.5)
  line L1904 (-101, -145) -> (-99, -145)
  line L1905 (-99, -145) -> (-99, -142.5)
  line L1906 (-101, -142.5) -> (-101, -145)
  line L1907 (-99, -142.5) -> (-101, -142.5)
  line L1908 (-111, -145) -> (-109, -145)
  line L1909 (-109, -145) -> (-109, -142.5)
  line L1910 (-111, -142.5) -> (-111, -145)
  line L1911 (-109, -142.5) -> (-111, -142.5)
  line L1912 (-121, -145) -> (-119, -145)
  line L1913 (-119, -145) -> (-119, -142.5)
  line L1914 (-121, -142.5) -> (-121, -145)
  line L1915 (-119, -142.5) -> (-121, -142.5)
  line L1916 (-131, -145) -> (-129, -145)
  line L1917 (-129, -145) -> (-129, -142.5)
  line L1918 (-131, -142.5) -> (-131, -145)
  line L1919 (-129, -142.5) -> (-131, -142.5)
  line L1920 (-141, -145) -> (-139, -145)
  line L1921 (-139, -145) -> (-139, -142.5)
  line L1922 (-141, -142.5) -> (-141, -145)
  line L1923 (-139, -142.5) -> (-141, -142.5)
  line L1924 (-151, -145) -> (-149, -145)
  line L1925 (-149, -145) -> (-149, -142.5)
  line L1926 (-151, -142.5) -> (-151, -145)
  line L1927 (-149, -142.5) -> (-151, -142.5)
  line L1928 (-11, -155) -> (-9, -155)
  line L1929 (-9, -155) -> (-9, -152.5)
  line L1930 (-11, -152.5) -> (-11, -155)
  line L1931 (-9, -152.5) -> (-11, -152.5)
  line L1932 (-21, -155) -> (-19, -155)
  line L1933 (-19, -155) -> (-19, -152.5)
  line L1934 (-21, -152.5) -> (-21, -155)
  line L1935 (-19, -152.5) -> (-21, -152.5)
  line L1936 (-31, -155) -> (-29, -155)
  line L1937 (-29, -155) -> (-29, -152.5)
  line L1938 (-31, -152.5) -> (-31, -155)
  line L1939 (-29, -152.5) -> (-31, -152.5)
  line L1940 (-41, -155) -> (-39, -155)
  line L1941 (-39, -155) -> (-39, -152.5)
  line L1942 (-41, -152.5) -> (-41, -155)
  line L1943 (-39, -152.5) -> (-41, -152.5)
  line L1944 (-51, -155) -> (-49, -155)
  line L1945 (-49, -155) -> (-49, -152.5)
  line L1946 (-51, -152.5) -> (-51, -155)
  line L1947 (-49, -152.5) -> (-51, -152.5)
  line L1948 (-61, -155) -> (-59, -155)
  line L1949 (-59, -155) -> (-59, -152.5)
  line L1950 (-61, -152.5) -> (-61, -155)
  line L1951 (-59, -152.5) -> (-61, -152.5)
  line L1952 (-71, -155) -> (-69, -155)
  line L1953 (-69, -155) -> (-69, -152.5)
  line L1954 (-71, -152.5) -> (-71, -155)
  line L1955 (-69, -152.5) -> (-71, -152.5)
  line L1956 (-81, -155) -> (-79, -155)
  line L1957 (-79, -155) -> (-79, -152.5)
  line L1958 (-81, -152.5) -> (-81, -155)
  line L1959 (-79, -152.5) -> (-81, -152.5)
  line L1960 (-91, -155) -> (-89, -155)
  line L1961 (-89, -155) -> (-89, -152.5)
  line L1962 (-91, -152.5) -> (-91, -155)
  line L1963 (-89, -152.5) -> (-91, -152.5)
  line L1964 (-101, -155) -> (-99, -155)
  line L1965 (-99, -155) -> (-99, -152.5)
  line L1966 (-101, -152.5) -> (-101, -155)
  line L1967 (-99, -152.5) -> (-101, -152.5)
  line L1968 (-111, -155) -> (-109, -155)
  line L1969 (-109, -155) -> (-109, -152.5)
  line L1970 (-111, -152.5) -> (-111, -155)
  line L1971 (-109, -152.5) -> (-111, -152.5)
  line L1972 (-121, -155) -> (-119, -155)
  line L1973 (-119, -155) -> (-119, -152.5)
  line L1974 (-121, -152.5) -> (-121, -155)
  line L1975 (-119, -152.5) -> (-121, -152.5)
  line L1976 (-131, -155) -> (-129, -155)
  line L1977 (-129, -155) -> (-129, -152.5)
  line L1978 (-131, -152.5) -> (-131, -155)
  line L1979 (-129, -152.5) -> (-131, -152.5)
  line L1980 (-141, -155) -> (-139, -155)
  line L1981 (-139, -155) -> (-139, -152.5)
  line L1982 (-141, -152.5) -> (-141, -155)
  line L1983 (-139, -152.5) -> (-141, -152.5)
  line L1984 (-151, -155) -> (-149, -155)
  line L1985 (-149, -155) -> (-149, -152.5)
  line L1986 (-151, -152.5) -> (-151, -155)
  line L1987 (-149, -152.5) -> (-151, -152.5)
  point P0 (-10, -2.5)
  dimension "d5" = 5
  dimension "d6" = 5
  dimension "d7" = 2.5
  dimension "d8" = 2.5
  dimension "d11" = -10
  dimension "d12" = -10
  dimension "d15" = 2
  dimension "d16" = 2.5
  dimension "d17" = 2.5
  dimension "d18" = 10
  dimension "d21" = -10
  dimension "d22" = -10
  constraint horizontal L4
  constraint vertical L5
  constraint horizontal L6
  constraint vertical L7
  constraint horizontal L1028
  constraint vertical L1029
  constraint horizontal L1030
  constraint vertical L1031
  constraint midpoint L1028 P0
  measures "d5" distance of L4.start L4.end
  measures "d6" distance of L4.start L6.end
  measures "d7" distance of L1 L4.start
  measures "d8" distance of L0 L4.start
  measures "d15" distance of L1028.start L1028.end
  measures "d16" distance of L1028.start L1030.end
  measures "d17" distance of L1 P0
  measures "d18" distance of L0 P0